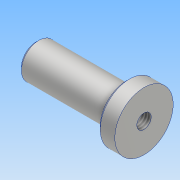
# Autodesk Inventor part: Pancake_Lever Mount Piece
Saved by Autodesk Inventor 2018.1 (Build 221171000, 171)
## iProperties
Created: 2019-02-14
Part Number: Pancake_Lever Mount Piece
Material: Aluminum 6061
Document SubType Name: Modeling
Designer: James
Density: 2.7 g/cm^3
Appearance: Aluminum - Flat
Author: James
Autodesk Inventor part; units mm, degrees
ref_plane "YZ Plane" through (0, 0, 0) normal (1, 0, 0) x (0, 1, 0)
ref_plane "XZ Plane" through (0, 0, 0) normal (0, 1, 0) x (-1, 0, 0)
ref_plane "XY Plane" through (0, 0, 0) normal (0, 0, 1) x (1, 0, 0)
sketch "Sketch1" plane through (0, 0, 0) normal (0, 0, 1) x (1, 0, 0)
  line L0 (0, 0) -> (15.5, 0)
  line L1 (15.5, 0) -> (15.5, 3)
  line L2 (15.5, 3) -> (0, 3)
  line L3 (0, 3) -> (0, 0)
  line L4 (15.5, 0) -> (18.5, 0)
  line L5 (18.5, 0) -> (18.5, 5)
  line L6 (18.5, 5) -> (15.5, 5)
  line L7 (15.5, 5) -> (15.5, 0)
  line L8 (0, 0) -> (18.5, 0)
  dimension "d0" = 5
  dimension "d1" = 3
  dimension "d2" = 15.5
  dimension "d3" = 3
  constraints: 18 end point, 4 parallel, 3 horizontal, 2 perpendicular
  measures "d0" distance between parallel lines of L4 L6
  measures "d1" distance of L2.end L0.start
  measures "d2" distance of L1.end L2.end
  measures "d3" distance of L5.end L6.end
revolve "Revolution1" add sketch "Sketch1" angle 360 about axis through (15.5, 0, 0) along (1, 0, 0)
fillet "Fillet1" radius 0.5 1 edges at (15.5, -3, 0)
chamfer "Chamfer1" distance 0.5 angle 45 2 edges at (0, -3, 0) (15.5, -5, 0)
sketch "Sketch2" plane through (18.5, 0, 0) normal (-1, 0, 0) x (0, 0, 1)
  circle A0 centre (0, 0) radius 3 projected
  point P0 (0, 0)
  constraints: 1 coincident
hole "Hole1" at (18.5, 0, 0) direction (-1, 0, 0) diameter 2.459 end through all thread size "M3x0.5" class "6H" standard "ANSI Metric M Profile"
body "Solid1"
